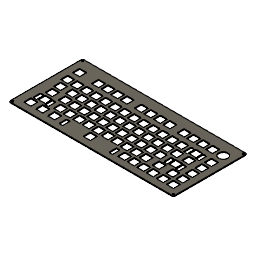
_Top_Mech_Case.fb088db0-0566-425f-93ac-fc1d6e48a953 (Autodesk Fusion 360 design; units mm, degrees)
part number: 2026-01-11-19-49-38-762
Autodesk Fusion 360 part; units mm, degrees
(part 1 of 3)
sketch "plate-2026-01-07T20_54_01.375Z" plane through (0, 0, 0) normal (0, 0, 1) x (1, 0, 0)
  line L0 (-11.2624, -135.013) -> (318.4436, -135.013)
  line L1 (318.4436, -135.013) -> (318.4436, 12.475)
  line L2 (318.4436, 12.475) -> (-11.2624, 12.475)
  line L3 (-11.2624, 12.475) -> (-11.2624, -135.013)
  line L4 (3.025, -7.287) -> (16.025, -7.287)
  line L5 (3.025, -21.287) -> (16.025, -21.287)
  line L6 (2.525, -7.787) -> (2.525, -20.787)
  line L7 (16.525, -7.787) -> (16.525, -20.787)
  arc A0 (3.025, -7.287) -> (2.525, -7.787) centre (3.025, -7.787) ccw
  arc A1 (16.525, -7.787) -> (16.025, -7.287) centre (16.025, -7.787) ccw
  arc A2 (2.525, -20.787) -> (3.025, -21.287) centre (3.025, -20.787) ccw
  arc A3 (16.025, -21.287) -> (16.525, -20.787) centre (16.025, -20.787) ccw
  line L8 (41.125, -7.287) -> (54.125, -7.287)
  line L9 (41.125, -21.287) -> (54.125, -21.287)
  line L10 (40.625, -7.787) -> (40.625, -20.787)
  line L11 (54.625, -7.787) -> (54.625, -20.787)
  arc A4 (41.125, -7.287) -> (40.625, -7.787) centre (41.125, -7.787) ccw
  arc A5 (54.625, -7.787) -> (54.125, -7.287) centre (54.125, -7.787) ccw
  arc A6 (40.625, -20.787) -> (41.125, -21.287) centre (41.125, -20.787) ccw
  arc A7 (54.125, -21.287) -> (54.625, -20.787) centre (54.125, -20.787) ccw
  line L12 (60.175, -7.287) -> (73.175, -7.287)
  line L13 (60.175, -21.287) -> (73.175, -21.287)
  line L14 (59.675, -7.787) -> (59.675, -20.787)
  line L15 (73.675, -7.787) -> (73.675, -20.787)
  arc A8 (60.175, -7.287) -> (59.675, -7.787) centre (60.175, -7.787) ccw
  arc A9 (73.675, -7.787) -> (73.175, -7.287) centre (73.175, -7.787) ccw
  arc A10 (59.675, -20.787) -> (60.175, -21.287) centre (60.175, -20.787) ccw
  arc A11 (73.175, -21.287) -> (73.675, -20.787) centre (73.175, -20.787) ccw
  line L16 (79.225, -7.287) -> (92.225, -7.287)
  line L17 (79.225, -21.287) -> (92.225, -21.287)
  line L18 (78.725, -7.787) -> (78.725, -20.787)
  line L19 (92.725, -7.787) -> (92.725, -20.787)
  arc A12 (79.225, -7.287) -> (78.725, -7.787) centre (79.225, -7.787) ccw
  arc A13 (92.725, -7.787) -> (92.225, -7.287) centre (92.225, -7.787) ccw
  arc A14 (78.725, -20.787) -> (79.225, -21.287) centre (79.225, -20.787) ccw
  arc A15 (92.225, -21.287) -> (92.725, -20.787) centre (92.225, -20.787) ccw
  line L20 (98.275, -7.287) -> (111.275, -7.287)
  line L21 (98.275, -21.287) -> (111.275, -21.287)
  line L22 (97.775, -7.787) -> (97.775, -20.787)
  line L23 (111.775, -7.787) -> (111.775, -20.787)
  arc A16 (98.275, -7.287) -> (97.775, -7.787) centre (98.275, -7.787) ccw
  arc A17 (111.775, -7.787) -> (111.275, -7.287) centre (111.275, -7.787) ccw
  arc A18 (97.775, -20.787) -> (98.275, -21.287) centre (98.275, -20.787) ccw
  arc A19 (111.275, -21.287) -> (111.775, -20.787) centre (111.275, -20.787) ccw
  line L24 (126.8501, -7.287) -> (139.8501, -7.287)
  line L25 (126.8501, -21.287) -> (139.8501, -21.287)
  line L26 (126.3501, -7.787) -> (126.3501, -20.787)
  line L27 (140.3501, -7.787) -> (140.3501, -20.787)
  arc A20 (126.8501, -7.287) -> (126.3501, -7.787) centre (126.8501, -7.787) ccw
  arc A21 (140.3501, -7.787) -> (139.8501, -7.287) centre (139.8501, -7.787) ccw
  arc A22 (126.3501, -20.787) -> (126.8501, -21.287) centre (126.8501, -20.787) ccw
  arc A23 (139.8501, -21.287) -> (140.3501, -20.787) centre (139.8501, -20.787) ccw
  line L28 (145.9001, -7.287) -> (158.9001, -7.287)
  line L29 (145.9001, -21.287) -> (158.9001, -21.287)
  line L30 (145.4001, -7.787) -> (145.4001, -20.787)
  line L31 (159.4001, -7.787) -> (159.4001, -20.787)
  arc A24 (145.9001, -7.287) -> (145.4001, -7.787) centre (145.9001, -7.787) ccw
  arc A25 (159.4001, -7.787) -> (158.9001, -7.287) centre (158.9001, -7.787) ccw
  arc A26 (145.4001, -20.787) -> (145.9001, -21.287) centre (145.9001, -20.787) ccw
  arc A27 (158.9001, -21.287) -> (159.4001, -20.787) centre (158.9001, -20.787) ccw
  line L32 (164.9501, -7.287) -> (177.9501, -7.287)
  line L33 (164.9501, -21.287) -> (177.9501, -21.287)
  line L34 (164.4501, -7.787) -> (164.4501, -20.787)
  line L35 (178.4501, -7.787) -> (178.4501, -20.787)
  arc A28 (164.9501, -7.287) -> (164.4501, -7.787) centre (164.9501, -7.787) ccw
  arc A29 (178.4501, -7.787) -> (177.9501, -7.287) centre (177.9501, -7.787) ccw
  arc A30 (164.4501, -20.787) -> (164.9501, -21.287) centre (164.9501, -20.787) ccw
  arc A31 (177.9501, -21.287) -> (178.4501, -20.787) centre (177.9501, -20.787) ccw
  line L36 (184.0001, -7.287) -> (197.0001, -7.287)
  line L37 (184.0001, -21.287) -> (197.0001, -21.287)
  line L38 (183.5001, -7.787) -> (183.5001, -20.787)
  line L39 (197.5001, -7.787) -> (197.5001, -20.787)
  arc A32 (184.0001, -7.287) -> (183.5001, -7.787) centre (184.0001, -7.787) ccw
  arc A33 (197.5001, -7.787) -> (197.0001, -7.287) centre (197.0001, -7.787) ccw
  arc A34 (183.5001, -20.787) -> (184.0001, -21.287) centre (184.0001, -20.787) ccw
  arc A35 (197.0001, -21.287) -> (197.5001, -20.787) centre (197.0001, -20.787) ccw
  line L40 (212.5752, -7.287) -> (225.5752, -7.287)
  line L41 (212.5752, -21.287) -> (225.5752, -21.287)
  line L42 (212.0752, -7.787) -> (212.0752, -20.787)
  line L43 (226.0752, -7.787) -> (226.0752, -20.787)
  arc A36 (212.5752, -7.287) -> (212.0752, -7.787) centre (212.5752, -7.787) ccw
  arc A37 (226.0752, -7.787) -> (225.5752, -7.287) centre (225.5752, -7.787) ccw
  arc A38 (212.0752, -20.787) -> (212.5752, -21.287) centre (212.5752, -20.787) ccw
  arc A39 (225.5752, -21.287) -> (226.0752, -20.787) centre (225.5752, -20.787) ccw
  line L44 (231.6252, -7.287) -> (244.6252, -7.287)
  line L45 (231.6253, -21.287) -> (244.6252, -21.287)
  line L46 (231.1252, -7.787) -> (231.1252, -20.787)
  line L47 (245.1252, -7.787) -> (245.1252, -20.787)
  arc A40 (231.6252, -7.287) -> (231.1252, -7.787) centre (231.6252, -7.787) ccw
  arc A41 (245.1252, -7.787) -> (244.6252, -7.287) centre (244.6252, -7.787) ccw
  arc A42 (231.1252, -20.787) -> (231.6253, -21.287) centre (231.6253, -20.787) ccw
  arc A43 (244.6252, -21.287) -> (245.1252, -20.787) centre (244.6252, -20.787) ccw
  line L48 (250.6752, -7.287) -> (263.6752, -7.287)
  line L49 (250.6753, -21.287) -> (263.6752, -21.287)
  line L50 (250.1752, -7.787) -> (250.1753, -20.787)
  line L51 (264.1753, -7.787) -> (264.1753, -20.787)
  arc A44 (250.6752, -7.287) -> (250.1752, -7.787) centre (250.6752, -7.787) ccw
  arc A45 (264.1753, -7.787) -> (263.6752, -7.287) centre (263.6752, -7.787) ccw
  arc A46 (250.1753, -20.787) -> (250.6753, -21.287) centre (250.6753, -20.787) ccw
  arc A47 (263.6752, -21.287) -> (264.1753, -20.787) centre (263.6752, -20.787) ccw
  line L52 (269.7253, -7.287) -> (282.7252, -7.287)
  line L53 (269.7253, -21.287) -> (282.7252, -21.287)
  line L54 (269.2252, -7.787) -> (269.2253, -20.787)
  line L55 (283.2253, -7.787) -> (283.2253, -20.787)
  arc A48 (269.7253, -7.287) -> (269.2252, -7.787) centre (269.7253, -7.787) ccw
  arc A49 (283.2253, -7.787) -> (282.7252, -7.287) centre (282.7252, -7.787) ccw
  arc A50 (269.2253, -20.787) -> (269.7253, -21.287) centre (269.7253, -20.787) ccw
  arc A51 (282.7252, -21.287) -> (283.2253, -20.787) centre (282.7252, -20.787) ccw
  line L56 (3.025, -31.1) -> (16.025, -31.1)
  line L57 (3.025, -45.1) -> (16.025, -45.1)
  line L58 (2.525, -31.6) -> (2.525, -44.6)
  line L59 (16.525, -31.6) -> (16.525, -44.6)
  arc A52 (3.025, -31.1) -> (2.525, -31.6) centre (3.025, -31.6) ccw
  arc A53 (16.525, -31.6) -> (16.025, -31.1) centre (16.025, -31.6) ccw
  arc A54 (2.525, -44.6) -> (3.025, -45.1) centre (3.025, -44.6) ccw
  arc A55 (16.025, -45.1) -> (16.525, -44.6) centre (16.025, -44.6) ccw
  line L60 (22.075, -31.1) -> (35.075, -31.1)
  line L61 (22.075, -45.1) -> (35.075, -45.1)
  line L62 (21.575, -31.6) -> (21.575, -44.6)
  line L63 (35.575, -31.6) -> (35.575, -44.6)
  arc A56 (22.075, -31.1) -> (21.575, -31.6) centre (22.075, -31.6) ccw
  arc A57 (35.575, -31.6) -> (35.075, -31.1) centre (35.075, -31.6) ccw
  arc A58 (21.575, -44.6) -> (22.075, -45.1) centre (22.075, -44.6) ccw
  arc A59 (35.075, -45.1) -> (35.575, -44.6) centre (35.075, -44.6) ccw
  line L64 (41.125, -31.1) -> (54.125, -31.1)
  line L65 (41.125, -45.1) -> (54.125, -45.1)
  line L66 (40.625, -31.6) -> (40.625, -44.6)
  line L67 (54.625, -31.6) -> (54.625, -44.6)
  arc A60 (41.125, -31.1) -> (40.625, -31.6) centre (41.125, -31.6) ccw
  arc A61 (54.625, -31.6) -> (54.125, -31.1) centre (54.125, -31.6) ccw
  arc A62 (40.625, -44.6) -> (41.125, -45.1) centre (41.125, -44.6) ccw
  arc A63 (54.125, -45.1) -> (54.625, -44.6) centre (54.125, -44.6) ccw
  line L68 (60.175, -31.1) -> (73.175, -31.1)
  line L69 (60.175, -45.1) -> (73.175, -45.1)
  line L70 (59.675, -31.6) -> (59.675, -44.6)
  line L71 (73.675, -31.6) -> (73.675, -44.6)
  arc A64 (60.175, -31.1) -> (59.675, -31.6) centre (60.175, -31.6) ccw
  arc A65 (73.675, -31.6) -> (73.175, -31.1) centre (73.175, -31.6) ccw
  arc A66 (59.675, -44.6) -> (60.175, -45.1) centre (60.175, -44.6) ccw
  arc A67 (73.175, -45.1) -> (73.675, -44.6) centre (73.175, -44.6) ccw
  line L72 (79.225, -31.1) -> (92.225, -31.1)
  line L73 (79.225, -45.1) -> (92.225, -45.1)
  line L74 (78.725, -31.6) -> (78.725, -44.6)
  line L75 (92.725, -31.6) -> (92.725, -44.6)
  arc A68 (79.225, -31.1) -> (78.725, -31.6) centre (79.225, -31.6) ccw
  arc A69 (92.725, -31.6) -> (92.225, -31.1) centre (92.225, -31.6) ccw
  arc A70 (78.725, -44.6) -> (79.225, -45.1) centre (79.225, -44.6) ccw
  arc A71 (92.225, -45.1) -> (92.725, -44.6) centre (92.225, -44.6) ccw
  line L76 (98.275, -31.1) -> (111.275, -31.1)
  line L77 (98.275, -45.1) -> (111.275, -45.1)
  line L78 (97.775, -31.6) -> (97.775, -44.6)
  line L79 (111.775, -31.6) -> (111.775, -44.6)
  arc A72 (98.275, -31.1) -> (97.775, -31.6) centre (98.275, -31.6) ccw
  arc A73 (111.775, -31.6) -> (111.275, -31.1) centre (111.275, -31.6) ccw
  arc A74 (97.775, -44.6) -> (98.275, -45.1) centre (98.275, -44.6) ccw
  arc A75 (111.275, -45.1) -> (111.775, -44.6) centre (111.275, -44.6) ccw
  line L80 (117.325, -31.1) -> (130.325, -31.1)
  line L81 (117.325, -45.1) -> (130.325, -45.1)
  line L82 (116.825, -31.6) -> (116.825, -44.6)
  line L83 (130.825, -31.6) -> (130.825, -44.6)
  arc A76 (117.325, -31.1) -> (116.825, -31.6) centre (117.325, -31.6) ccw
  arc A77 (130.825, -31.6) -> (130.325, -31.1) centre (130.325, -31.6) ccw
  arc A78 (116.825, -44.6) -> (117.325, -45.1) centre (117.325, -44.6) ccw
  arc A79 (130.325, -45.1) -> (130.825, -44.6) centre (130.325, -44.6) ccw
  line L84 (136.375, -31.1) -> (149.375, -31.1)
  line L85 (136.375, -45.1) -> (149.375, -45.1)
  line L86 (135.875, -31.6) -> (135.875, -44.6)
  line L87 (149.875, -31.6) -> (149.875, -44.6)
  arc A80 (136.375, -31.1) -> (135.875, -31.6) centre (136.375, -31.6) ccw
  arc A81 (149.875, -31.6) -> (149.375, -31.1) centre (149.375, -31.6) ccw
  arc A82 (135.875, -44.6) -> (136.375, -45.1) centre (136.375, -44.6) ccw
  arc A83 (149.375, -45.1) -> (149.875, -44.6) centre (149.375, -44.6) ccw
  line L88 (155.425, -31.1) -> (168.425, -31.1)
  line L89 (155.425, -45.1) -> (168.425, -45.1)
  line L90 (154.925, -31.6) -> (154.925, -44.6)
  line L91 (168.925, -31.6) -> (168.925, -44.6)
  arc A84 (155.425, -31.1) -> (154.925, -31.6) centre (155.425, -31.6) ccw
  arc A85 (168.925, -31.6) -> (168.425, -31.1) centre (168.425, -31.6) ccw
  arc A86 (154.925, -44.6) -> (155.425, -45.1) centre (155.425, -44.6) ccw
  arc A87 (168.425, -45.1) -> (168.925, -44.6) centre (168.425, -44.6) ccw
  line L92 (174.475, -31.1) -> (187.475, -31.1)
  line L93 (174.475, -45.1) -> (187.475, -45.1)
  line L94 (173.975, -31.6) -> (173.975, -44.6)
  line L95 (187.975, -31.6) -> (187.975, -44.6)
  arc A88 (174.475, -31.1) -> (173.975, -31.6) centre (174.475, -31.6) ccw
  arc A89 (187.975, -31.6) -> (187.475, -31.1) centre (187.475, -31.6) ccw
  arc A90 (173.975, -44.6) -> (174.475, -45.1) centre (174.475, -44.6) ccw
  arc A91 (187.475, -45.1) -> (187.975, -44.6) centre (187.475, -44.6) ccw
  line L96 (193.525, -31.1) -> (206.525, -31.1)
  line L97 (193.525, -45.1) -> (206.525, -45.1)
  line L98 (193.025, -31.6) -> (193.025, -44.6)
  line L99 (207.025, -31.6) -> (207.025, -44.6)
  arc A92 (193.525, -31.1) -> (193.025, -31.6) centre (193.525, -31.6) ccw
  arc A93 (207.025, -31.6) -> (206.525, -31.1) centre (206.525, -31.6) ccw
  arc A94 (193.025, -44.6) -> (193.525, -45.1) centre (193.525, -44.6) ccw
  arc A95 (206.525, -45.1) -> (207.025, -44.6) centre (206.525, -44.6) ccw
  line L100 (212.575, -31.1) -> (225.575, -31.1)
  line L101 (212.575, -45.1) -> (225.575, -45.1)
  line L102 (212.075, -31.6) -> (212.075, -44.6)
  line L103 (226.075, -31.6) -> (226.075, -44.6)
  arc A96 (212.575, -31.1) -> (212.075, -31.6) centre (212.575, -31.6) ccw
  arc A97 (226.075, -31.6) -> (225.575, -31.1) centre (225.575, -31.6) ccw
  arc A98 (212.075, -44.6) -> (212.575, -45.1) centre (212.575, -44.6) ccw
  arc A99 (225.575, -45.1) -> (226.075, -44.6) centre (225.575, -44.6) ccw
  line L104 (231.625, -31.1) -> (244.625, -31.1)
  line L105 (231.625, -45.1) -> (244.625, -45.1)
  line L106 (231.125, -31.6) -> (231.125, -44.6)
  line L107 (245.125, -31.6) -> (245.125, -44.6)
  arc A100 (231.625, -31.1) -> (231.125, -31.6) centre (231.625, -31.6) ccw
  arc A101 (245.125, -31.6) -> (244.625, -31.1) centre (244.625, -31.6) ccw
  arc A102 (231.125, -44.6) -> (231.625, -45.1) centre (231.625, -44.6) ccw
  arc A103 (244.625, -45.1) -> (245.125, -44.6) centre (244.625, -44.6) ccw
  line L108 (260.2, -31.1) -> (273.2, -31.1)
  line L109 (260.2, -45.1) -> (273.2, -45.1)
  line L110 (259.7, -31.6) -> (259.7, -44.6)
  line L111 (273.7, -31.6) -> (273.7, -44.6)
  arc A104 (260.2, -31.1) -> (259.7, -31.6) centre (260.2, -31.6) ccw
  arc A105 (273.7, -31.6) -> (273.2, -31.1) centre (273.2, -31.6) ccw
  arc A106 (259.7, -44.6) -> (260.2, -45.1) centre (260.2, -44.6) ccw
  arc A107 (273.2, -45.1) -> (273.7, -44.6) centre (273.2, -44.6) ccw
  line L112 (251.762, -32.1) -> (257.762, -32.1)
  line L113 (251.762, -47.1) -> (257.762, -47.1)
  line L114 (251.262, -32.6) -> (251.262, -46.6)
  line L115 (258.262, -32.6) -> (258.262, -46.6)
  arc A108 (251.762, -32.1) -> (251.262, -32.6) centre (251.762, -32.6) ccw
  arc A109 (258.262, -32.6) -> (257.762, -32.1) centre (257.762, -32.6) ccw
  arc A110 (251.262, -46.6) -> (251.762, -47.1) centre (251.762, -46.6) ccw
  arc A111 (257.762, -47.1) -> (258.262, -46.6) centre (257.762, -46.6) ccw
  line L116 (275.638, -32.1) -> (281.638, -32.1)
  line L117 (275.638, -47.1) -> (281.638, -47.1)
  line L118 (275.138, -32.6) -> (275.138, -46.6)
  line L119 (282.138, -32.6) -> (282.138, -46.6)
  arc A112 (275.638, -32.1) -> (275.138, -32.6) centre (275.638, -32.6) ccw
  arc A113 (282.138, -32.6) -> (281.638, -32.1) centre (281.638, -32.6) ccw
  arc A114 (275.138, -46.6) -> (275.638, -47.1) centre (275.638, -46.6) ccw
  arc A115 (281.638, -47.1) -> (282.138, -46.6) centre (281.638, -46.6) ccw
  line L120 (291.1562, -31.1) -> (304.1562, -31.1)
  line L121 (291.1562, -45.1) -> (304.1562, -45.1)
  line L122 (290.6562, -31.6) -> (290.6562, -44.6)
  line L123 (304.6562, -31.6) -> (304.6562, -44.6)
  arc A116 (291.1562, -31.1) -> (290.6562, -31.6) centre (291.1562, -31.6) ccw
  arc A117 (304.6562, -31.6) -> (304.1562, -31.1) centre (304.1562, -31.6) ccw
  arc A118 (290.6562, -44.6) -> (291.1562, -45.1) centre (291.1562, -44.6) ccw
  arc A119 (304.1562, -45.1) -> (304.6562, -44.6) centre (304.1562, -44.6) ccw
  line L124 (7.7875, -50.15) -> (20.7875, -50.15)
  line L125 (7.7875, -64.15) -> (20.7875, -64.15)
  line L126 (7.2875, -50.65) -> (7.2875, -63.65)
  line L127 (21.2875, -50.65) -> (21.2875, -63.65)
  arc A120 (7.7875, -50.15) -> (7.2875, -50.65) centre (7.7875, -50.65) ccw
  arc A121 (21.2875, -50.65) -> (20.7875, -50.15) centre (20.7875, -50.65) ccw
  arc A122 (7.2875, -63.65) -> (7.7875, -64.15) centre (7.7875, -63.65) ccw
  arc A123 (20.7875, -64.15) -> (21.2875, -63.65) centre (20.7875, -63.65) ccw
  line L128 (31.6, -50.15) -> (44.6, -50.15)
  line L129 (31.6, -64.15) -> (44.6, -64.15)
  line L130 (31.1, -50.65) -> (31.1, -63.65)
  line L131 (45.1, -50.65) -> (45.1, -63.65)
  arc A124 (31.6, -50.15) -> (31.1, -50.65) centre (31.6, -50.65) ccw
  arc A125 (45.1, -50.65) -> (44.6, -50.15) centre (44.6, -50.65) ccw
  arc A126 (31.1, -63.65) -> (31.6, -64.15) centre (31.6, -63.65) ccw
  arc A127 (44.6, -64.15) -> (45.1, -63.65) centre (44.6, -63.65) ccw
  line L132 (50.65, -50.15) -> (63.65, -50.15)
  line L133 (50.65, -64.15) -> (63.65, -64.15)
  line L134 (50.15, -50.65) -> (50.15, -63.65)
  line L135 (64.15, -50.65) -> (64.15, -63.65)
  arc A128 (50.65, -50.15) -> (50.15, -50.65) centre (50.65, -50.65) ccw
  arc A129 (64.15, -50.65) -> (63.65, -50.15) centre (63.65, -50.65) ccw
  arc A130 (50.15, -63.65) -> (50.65, -64.15) centre (50.65, -63.65) ccw
  arc A131 (63.65, -64.15) -> (64.15, -63.65) centre (63.65, -63.65) ccw
  line L136 (69.7, -50.15) -> (82.7, -50.15)
  line L137 (69.7, -64.15) -> (82.7, -64.15)
  line L138 (69.2, -50.65) -> (69.2, -63.65)
  line L139 (83.2, -50.65) -> (83.2, -63.65)
  arc A132 (69.7, -50.15) -> (69.2, -50.65) centre (69.7, -50.65) ccw
  arc A133 (83.2, -50.65) -> (82.7, -50.15) centre (82.7, -50.65) ccw
  arc A134 (69.2, -63.65) -> (69.7, -64.15) centre (69.7, -63.65) ccw
  arc A135 (82.7, -64.15) -> (83.2, -63.65) centre (82.7, -63.65) ccw
  line L140 (88.75, -50.15) -> (101.75, -50.15)
  line L141 (88.75, -64.15) -> (101.75, -64.15)
  line L142 (88.25, -50.65) -> (88.25, -63.65)
  line L143 (102.25, -50.65) -> (102.25, -63.65)
  arc A136 (88.75, -50.15) -> (88.25, -50.65) centre (88.75, -50.65) ccw
  arc A137 (102.25, -50.65) -> (101.75, -50.15) centre (101.75, -50.65) ccw
  arc A138 (88.25, -63.65) -> (88.75, -64.15) centre (88.75, -63.65) ccw
  arc A139 (101.75, -64.15) -> (102.25, -63.65) centre (101.75, -63.65) ccw
  line L144 (107.8, -50.15) -> (120.8, -50.15)
  line L145 (107.8, -64.15) -> (120.8, -64.15)
  line L146 (107.3, -50.65) -> (107.3, -63.65)
  line L147 (121.3, -50.65) -> (121.3, -63.65)
  arc A140 (107.8, -50.15) -> (107.3, -50.65) centre (107.8, -50.65) ccw
  arc A141 (121.3, -50.65) -> (120.8, -50.15) centre (120.8, -50.65) ccw
  arc A142 (107.3, -63.65) -> (107.8, -64.15) centre (107.8, -63.65) ccw
  arc A143 (120.8, -64.15) -> (121.3, -63.65) centre (120.8, -63.65) ccw
  line L148 (126.85, -50.15) -> (139.85, -50.15)
  line L149 (126.85, -64.15) -> (139.85, -64.15)
  line L150 (126.35, -50.65) -> (126.35, -63.65)
  line L151 (140.35, -50.65) -> (140.35, -63.65)
  arc A144 (126.85, -50.15) -> (126.35, -50.65) centre (126.85, -50.65) ccw
  arc A145 (140.35, -50.65) -> (139.85, -50.15) centre (139.85, -50.65) ccw
  arc A146 (126.35, -63.65) -> (126.85, -64.15) centre (126.85, -63.65) ccw
  arc A147 (139.85, -64.15) -> (140.35, -63.65) centre (139.85, -63.65) ccw
  line L152 (145.9, -50.15) -> (158.9, -50.15)
  line L153 (145.9, -64.15) -> (158.9, -64.15)
  line L154 (145.4, -50.65) -> (145.4, -63.65)
  line L155 (159.4, -50.65) -> (159.4, -63.65)
  arc A148 (145.9, -50.15) -> (145.4, -50.65) centre (145.9, -50.65) ccw
  arc A149 (159.4, -50.65) -> (158.9, -50.15) centre (158.9, -50.65) ccw
  arc A150 (145.4, -63.65) -> (145.9, -64.15) centre (145.9, -63.65) ccw
  arc A151 (158.9, -64.15) -> (159.4, -63.65) centre (158.9, -63.65) ccw
  line L156 (164.95, -50.15) -> (177.95, -50.15)
  line L157 (164.95, -64.15) -> (177.95, -64.15)
  line L158 (164.45, -50.65) -> (164.45, -63.65)
  line L159 (178.45, -50.65) -> (178.45, -63.65)
  arc A152 (164.95, -50.15) -> (164.45, -50.65) centre (164.95, -50.65) ccw
  arc A153 (178.45, -50.65) -> (177.95, -50.15) centre (177.95, -50.65) ccw
  arc A154 (164.45, -63.65) -> (164.95, -64.15) centre (164.95, -63.65) ccw
  arc A155 (177.95, -64.15) -> (178.45, -63.65) centre (177.95, -63.65) ccw
  line L160 (184, -50.15) -> (197, -50.15)
  line L161 (184, -64.15) -> (197, -64.15)
  line L162 (183.5, -50.65) -> (183.5, -63.65)
  line L163 (197.5, -50.65) -> (197.5, -63.65)
  arc A156 (184, -50.15) -> (183.5, -50.65) centre (184, -50.65) ccw
  arc A157 (197.5, -50.65) -> (197, -50.15) centre (197, -50.65) ccw
  arc A158 (183.5, -63.65) -> (184, -64.15) centre (184, -63.65) ccw
  arc A159 (197, -64.15) -> (197.5, -63.65) centre (197, -63.65) ccw
  line L164 (203.05, -50.15) -> (216.05, -50.15)
  line L165 (203.05, -64.15) -> (216.05, -64.15)
  line L166 (202.55, -50.65) -> (202.55, -63.65)
  line L167 (216.55, -50.65) -> (216.55, -63.65)
  arc A160 (203.05, -50.15) -> (202.55, -50.65) centre (203.05, -50.65) ccw
  arc A161 (216.55, -50.65) -> (216.05, -50.15) centre (216.05, -50.65) ccw
  arc A162 (202.55, -63.65) -> (203.05, -64.15) centre (203.05, -63.65) ccw
  arc A163 (216.05, -64.15) -> (216.55, -63.65) centre (216.05, -63.65) ccw
  line L168 (222.1, -50.15) -> (235.1, -50.15)
  line L169 (222.1, -64.15) -> (235.1, -64.15)
  line L170 (221.6, -50.65) -> (221.6, -63.65)
  line L171 (235.6, -50.65) -> (235.6, -63.65)
  arc A164 (222.1, -50.15) -> (221.6, -50.65) centre (222.1, -50.65) ccw
  arc A165 (235.6, -50.65) -> (235.1, -50.15) centre (235.1, -50.65) ccw
  arc A166 (221.6, -63.65) -> (222.1, -64.15) centre (222.1, -63.65) ccw
  arc A167 (235.1, -64.15) -> (235.6, -63.65) centre (235.1, -63.65) ccw
  line L172 (241.15, -50.15) -> (254.15, -50.15)
  line L173 (241.15, -64.15) -> (254.15, -64.15)
  line L174 (240.65, -50.65) -> (240.65, -63.65)
  line L175 (254.65, -50.65) -> (254.65, -63.65)
  arc A168 (241.15, -50.15) -> (240.65, -50.65) centre (241.15, -50.65) ccw
  arc A169 (254.65, -50.65) -> (254.15, -50.15) centre (254.15, -50.65) ccw
  arc A170 (240.65, -63.65) -> (241.15, -64.15) centre (241.15, -63.65) ccw
  arc A171 (254.15, -64.15) -> (254.65, -63.65) centre (254.15, -63.65) ccw
  line L176 (264.9625, -50.15) -> (277.9625, -50.15)
  line L177 (264.9625, -64.15) -> (277.9625, -64.15)
  line L178 (264.4625, -50.65) -> (264.4625, -63.65)
  line L179 (278.4625, -50.65) -> (278.4625, -63.65)
  arc A172 (264.9625, -50.15) -> (264.4625, -50.65) centre (264.9625, -50.65) ccw
  arc A173 (278.4625, -50.65) -> (277.9625, -50.15) centre (277.9625, -50.65) ccw
  arc A174 (264.4625, -63.65) -> (264.9625, -64.15) centre (264.9625, -63.65) ccw
  arc A175 (277.9625, -64.15) -> (278.4625, -63.65) centre (277.9625, -63.65) ccw
  line L180 (291.1562, -50.15) -> (304.1562, -50.15)
  line L181 (291.1562, -64.15) -> (304.1562, -64.15)
  line L182 (290.6562, -50.65) -> (290.6562, -63.65)
  line L183 (304.6562, -50.65) -> (304.6562, -63.65)
  arc A176 (291.1562, -50.15) -> (290.6562, -50.65) centre (291.1562, -50.65) ccw
  arc A177 (304.6562, -50.65) -> (304.1562, -50.15) centre (304.1562, -50.65) ccw
  arc A178 (290.6562, -63.65) -> (291.1562, -64.15) centre (291.1562, -63.65) ccw
  arc A179 (304.1562, -64.15) -> (304.6562, -63.65) centre (304.1562, -63.65) ccw
  line L184 (10.1687, -69.2) -> (23.1687, -69.2)
  line L185 (10.1687, -83.2) -> (23.1687, -83.2)
  line L186 (9.6687, -69.7) -> (9.6687, -82.7)
  line L187 (23.6687, -69.7) -> (23.6687, -82.7)
  arc A180 (10.1687, -69.2) -> (9.6688, -69.7) centre (10.1687, -69.7) ccw
  arc A181 (23.6687, -69.7) -> (23.1687, -69.2) centre (23.1687, -69.7) ccw
  arc A182 (9.6687, -82.7) -> (10.1687, -83.2) centre (10.1687, -82.7) ccw
  arc A183 (23.1687, -83.2) -> (23.6687, -82.7) centre (23.1687, -82.7) ccw
  line L188 (36.3625, -69.2) -> (49.3625, -69.2)
  line L189 (36.3625, -83.2) -> (49.3625, -83.2)
  line L190 (35.8625, -69.7) -> (35.8625, -82.7)
  line L191 (49.8625, -69.7) -> (49.8625, -82.7)
  arc A184 (36.3625, -69.2) -> (35.8625, -69.7) centre (36.3625, -69.7) ccw
  arc A185 (49.8625, -69.7) -> (49.3625, -69.2) centre (49.3625, -69.7) ccw
  arc A186 (35.8625, -82.7) -> (36.3625, -83.2) centre (36.3625, -82.7) ccw
  arc A187 (49.3625, -83.2) -> (49.8625, -82.7) centre (49.3625, -82.7) ccw
  line L192 (55.4125, -69.2) -> (68.4125, -69.2)
  line L193 (55.4125, -83.2) -> (68.4125, -83.2)
  line L194 (54.9125, -69.7) -> (54.9125, -82.7)
  line L195 (68.9125, -69.7) -> (68.9125, -82.7)
  arc A188 (55.4125, -69.2) -> (54.9125, -69.7) centre (55.4125, -69.7) ccw
  arc A189 (68.9125, -69.7) -> (68.4125, -69.2) centre (68.4125, -69.7) ccw
  arc A190 (54.9125, -82.7) -> (55.4125, -83.2) centre (55.4125, -82.7) ccw
  arc A191 (68.4125, -83.2) -> (68.9125, -82.7) centre (68.4125, -82.7) ccw
  line L196 (74.4625, -69.2) -> (87.4625, -69.2)
  line L197 (74.4625, -83.2) -> (87.4625, -83.2)
  line L198 (73.9625, -69.7) -> (73.9625, -82.7)
  line L199 (87.9625, -69.7) -> (87.9625, -82.7)
  arc A192 (74.4625, -69.2) -> (73.9625, -69.7) centre (74.4625, -69.7) ccw
  arc A193 (87.9625, -69.7) -> (87.4625, -69.2) centre (87.4625, -69.7) ccw
  arc A194 (73.9625, -82.7) -> (74.4625, -83.2) centre (74.4625, -82.7) ccw
  arc A195 (87.4625, -83.2) -> (87.9625, -82.7) centre (87.4625, -82.7) ccw
  line L200 (93.5125, -69.2) -> (106.5125, -69.2)
  line L201 (93.5125, -83.2) -> (106.5125, -83.2)
  line L202 (93.0125, -69.7) -> (93.0125, -82.7)
  line L203 (107.0125, -69.7) -> (107.0125, -82.7)
  arc A196 (93.5125, -69.2) -> (93.0125, -69.7) centre (93.5125, -69.7) ccw
  arc A197 (107.0125, -69.7) -> (106.5125, -69.2) centre (106.5125, -69.7) ccw
  arc A198 (93.0125, -82.7) -> (93.5125, -83.2) centre (93.5125, -82.7) ccw
  arc A199 (106.5125, -83.2) -> (107.0125, -82.7) centre (106.5125, -82.7) ccw
  line L204 (112.5625, -69.2) -> (125.5625, -69.2)
  line L205 (112.5625, -83.2) -> (125.5625, -83.2)
  line L206 (112.0625, -69.7) -> (112.0625, -82.7)
  line L207 (126.0625, -69.7) -> (126.0625, -82.7)
  arc A200 (112.5625, -69.2) -> (112.0625, -69.7) centre (112.5625, -69.7) ccw
  arc A201 (126.0625, -69.7) -> (125.5625, -69.2) centre (125.5625, -69.7) ccw
  arc A202 (112.0625, -82.7) -> (112.5625, -83.2) centre (112.5625, -82.7) ccw
  arc A203 (125.5625, -83.2) -> (126.0625, -82.7) centre (125.5625, -82.7) ccw
  line L208 (131.6125, -69.2) -> (144.6125, -69.2)
  line L209 (131.6125, -83.2) -> (144.6125, -83.2)
  line L210 (131.1125, -69.7) -> (131.1125, -82.7)
  line L211 (145.1125, -69.7) -> (145.1125, -82.7)
  arc A204 (131.6125, -69.2) -> (131.1125, -69.7) centre (131.6125, -69.7) ccw
  arc A205 (145.1125, -69.7) -> (144.6125, -69.2) centre (144.6125, -69.7) ccw
  arc A206 (131.1125, -82.7) -> (131.6125, -83.2) centre (131.6125, -82.7) ccw
  arc A207 (144.6125, -83.2) -> (145.1125, -82.7) centre (144.6125, -82.7) ccw
  line L212 (150.6625, -69.2) -> (163.6625, -69.2)
  line L213 (150.6625, -83.2) -> (163.6625, -83.2)
  line L214 (150.1625, -69.7) -> (150.1625, -82.7)
  line L215 (164.1625, -69.7) -> (164.1625, -82.7)
  arc A208 (150.6625, -69.2) -> (150.1625, -69.7) centre (150.6625, -69.7) ccw
  arc A209 (164.1625, -69.7) -> (163.6625, -69.2) centre (163.6625, -69.7) ccw
  arc A210 (150.1625, -82.7) -> (150.6625, -83.2) centre (150.6625, -82.7) ccw
  arc A211 (163.6625, -83.2) -> (164.1625, -82.7) centre (163.6625, -82.7) ccw
  line L216 (169.7125, -69.2) -> (182.7125, -69.2)
  line L217 (169.7125, -83.2) -> (182.7125, -83.2)
  line L218 (169.2125, -69.7) -> (169.2125, -82.7)
  line L219 (183.2125, -69.7) -> (183.2125, -82.7)
  arc A212 (169.7125, -69.2) -> (169.2125, -69.7) centre (169.7125, -69.7) ccw
  arc A213 (183.2125, -69.7) -> (182.7125, -69.2) centre (182.7125, -69.7) ccw
  arc A214 (169.2125, -82.7) -> (169.7125, -83.2) centre (169.7125, -82.7) ccw
  arc A215 (182.7125, -83.2) -> (183.2125, -82.7) centre (182.7125, -82.7) ccw
  line L220 (188.7625, -69.2) -> (201.7625, -69.2)
  line L221 (188.7625, -83.2) -> (201.7625, -83.2)
  line L222 (188.2625, -69.7) -> (188.2625, -82.7)
  line L223 (202.2625, -69.7) -> (202.2625, -82.7)
  arc A216 (188.7625, -69.2) -> (188.2625, -69.7) centre (188.7625, -69.7) ccw
  arc A217 (202.2625, -69.7) -> (201.7625, -69.2) centre (201.7625, -69.7) ccw
  arc A218 (188.2625, -82.7) -> (188.7625, -83.2) centre (188.7625, -82.7) ccw
  arc A219 (201.7625, -83.2) -> (202.2625, -82.7) centre (201.7625, -82.7) ccw
  line L224 (207.8125, -69.2) -> (220.8125, -69.2)
  line L225 (207.8125, -83.2) -> (220.8125, -83.2)
  line L226 (207.3125, -69.7) -> (207.3125, -82.7)
  line L227 (221.3125, -69.7) -> (221.3125, -82.7)
  arc A220 (207.8125, -69.2) -> (207.3125, -69.7) centre (207.8125, -69.7) ccw
  arc A221 (221.3125, -69.7) -> (220.8125, -69.2) centre (220.8125, -69.7) ccw
  arc A222 (207.3125, -82.7) -> (207.8125, -83.2) centre (207.8125, -82.7) ccw
  arc A223 (220.8125, -83.2) -> (221.3125, -82.7) centre (220.8125, -82.7) ccw
  line L228 (226.8625, -69.2) -> (239.8625, -69.2)
  line L229 (226.8625, -83.2) -> (239.8625, -83.2)
  line L230 (226.3625, -69.7) -> (226.3625, -82.7)
  line L231 (240.3625, -69.7) -> (240.3625, -82.7)
  arc A224 (226.8625, -69.2) -> (226.3625, -69.7) centre (226.8625, -69.7) ccw
  arc A225 (240.3625, -69.7) -> (239.8625, -69.2) centre (239.8625, -69.7) ccw
  arc A226 (226.3625, -82.7) -> (226.8625, -83.2) centre (226.8625, -82.7) ccw
  arc A227 (239.8625, -83.2) -> (240.3625, -82.7) centre (239.8625, -82.7) ccw
  line L232 (257.8188, -69.2) -> (270.8188, -69.2)
  line L233 (257.8188, -83.2) -> (270.8188, -83.2)
  line L234 (257.3188, -69.7) -> (257.3188, -82.7)
  line L235 (271.3188, -69.7) -> (271.3188, -82.7)
  arc A228 (257.8188, -69.2) -> (257.3188, -69.7) centre (257.8188, -69.7) ccw
  arc A229 (271.3188, -69.7) -> (270.8188, -69.2) centre (270.8188, -69.7) ccw
  arc A230 (257.3188, -82.7) -> (257.8188, -83.2) centre (257.8188, -82.7) ccw
  arc A231 (270.8188, -83.2) -> (271.3188, -82.7) centre (270.8188, -82.7) ccw
  line L236 (249.3808, -70.2) -> (255.3808, -70.2)
  line L237 (249.3808, -85.2) -> (255.3808, -85.2)
  line L238 (248.8808, -70.7) -> (248.8808, -84.7)
  line L239 (255.8808, -70.7) -> (255.8808, -84.7)
  arc A232 (249.3808, -70.2) -> (248.8808, -70.7) centre (249.3808, -70.7) ccw
  arc A233 (255.8808, -70.7) -> (255.3808, -70.2) centre (255.3808, -70.7) ccw
  arc A234 (248.8808, -84.7) -> (249.3808, -85.2) centre (249.3808, -84.7) ccw
  arc A235 (255.3808, -85.2) -> (255.8808, -84.7) centre (255.3808, -84.7) ccw
  line L240 (273.2568, -70.2) -> (279.2568, -70.2)
  line L241 (273.2568, -85.2) -> (279.2568, -85.2)
  line L242 (272.7568, -70.7) -> (272.7568, -84.7)
  line L243 (279.7568, -70.7) -> (279.7568, -84.7)
  arc A236 (273.2568, -70.2) -> (272.7568, -70.7) centre (273.2568, -70.7) ccw
  arc A237 (279.7568, -70.7) -> (279.2568, -70.2) centre (279.2568, -70.7) ccw
  arc A238 (272.7568, -84.7) -> (273.2568, -85.2) centre (273.2568, -84.7) ccw
  arc A239 (279.2568, -85.2) -> (279.7568, -84.7) centre (279.2568, -84.7) ccw
  line L244 (291.1562, -69.2) -> (304.1562, -69.2)
  line L245 (291.1562, -83.2) -> (304.1562, -83.2)
  line L246 (290.6562, -69.7) -> (290.6562, -82.7)
  line L247 (304.6562, -69.7) -> (304.6562, -82.7)
  arc A240 (291.1562, -69.2) -> (290.6562, -69.7) centre (291.1562, -69.7) ccw
  arc A241 (304.6562, -69.7) -> (304.1562, -69.2) centre (304.1562, -69.7) ccw
  arc A242 (290.6562, -82.7) -> (291.1562, -83.2) centre (291.1562, -82.7) ccw
  arc A243 (304.1562, -83.2) -> (304.6562, -82.7) centre (304.1562, -82.7) ccw
  line L248 (14.9313, -88.25) -> (27.9312, -88.25)
  line L249 (14.9313, -102.25) -> (27.9312, -102.25)
  line L250 (14.4313, -88.75) -> (14.4313, -101.75)
  line L251 (28.4313, -88.75) -> (28.4313, -101.75)
  arc A244 (14.9313, -88.25) -> (14.4313, -88.75) centre (14.9313, -88.75) ccw
  arc A245 (28.4313, -88.75) -> (27.9312, -88.25) centre (27.9312, -88.75) ccw
  arc A246 (14.4313, -101.75) -> (14.9313, -102.25) centre (14.9313, -101.75) ccw
  arc A247 (27.9312, -102.25) -> (28.4313, -101.75) centre (27.9312, -101.75) ccw
  line L252 (6.4933, -89.25) -> (12.4932, -89.25)
  line L253 (6.4933, -104.25) -> (12.4932, -104.25)
  line L254 (5.9932, -89.75) -> (5.9932, -103.75)
  line L255 (12.9932, -89.75) -> (12.9932, -103.75)
  arc A248 (6.4933, -89.25) -> (5.9933, -89.75) centre (6.4933, -89.75) ccw
  arc A249 (12.9932, -89.75) -> (12.4932, -89.25) centre (12.4932, -89.75) ccw
  arc A250 (5.9932, -103.75) -> (6.4933, -104.25) centre (6.4933, -103.75) ccw
  arc A251 (12.4932, -104.25) -> (12.9933, -103.75) centre (12.4932, -103.75) ccw
  line L256 (30.3693, -89.25) -> (36.3693, -89.25)
  line L257 (30.3693, -104.25) -> (36.3693, -104.25)
  line L258 (29.8693, -89.75) -> (29.8693, -103.75)
  line L259 (36.8693, -89.75) -> (36.8693, -103.75)
  arc A252 (30.3693, -89.25) -> (29.8693, -89.75) centre (30.3693, -89.75) ccw
  arc A253 (36.8693, -89.75) -> (36.3693, -89.25) centre (36.3693, -89.75) ccw
  arc A254 (29.8693, -103.75) -> (30.3693, -104.25) centre (30.3693, -103.75) ccw
  arc A255 (36.3693, -104.25) -> (36.8693, -103.75) centre (36.3693, -103.75) ccw
  line L260 (45.8875, -88.25) -> (58.8875, -88.25)
  line L261 (45.8875, -102.25) -> (58.8875, -102.25)
  line L262 (45.3875, -88.75) -> (45.3875, -101.75)
  line L263 (59.3875, -88.75) -> (59.3875, -101.75)
  arc A256 (45.8875, -88.25) -> (45.3875, -88.75) centre (45.8875, -88.75) ccw
  arc A257 (59.3875, -88.75) -> (58.8875, -88.25) centre (58.8875, -88.75) ccw
  arc A258 (45.3875, -101.75) -> (45.8875, -102.25) centre (45.8875, -101.75) ccw
  arc A259 (58.8875, -102.25) -> (59.3875, -101.75) centre (58.8875, -101.75) ccw
  line L264 (64.9375, -88.25) -> (77.9375, -88.25)
  line L265 (64.9375, -102.25) -> (77.9375, -102.25)
  line L266 (64.4375, -88.75) -> (64.4375, -101.75)
  line L267 (78.4375, -88.75) -> (78.4375, -101.75)
  arc A260 (64.9375, -88.25) -> (64.4375, -88.75) centre (64.9375, -88.75) ccw
  arc A261 (78.4375, -88.75) -> (77.9375, -88.25) centre (77.9375, -88.75) ccw
  arc A262 (64.4375, -101.75) -> (64.9375, -102.25) centre (64.9375, -101.75) ccw
  arc A263 (77.9375, -102.25) -> (78.4375, -101.75) centre (77.9375, -101.75) ccw
  line L268 (83.9875, -88.25) -> (96.9875, -88.25)
  line L269 (83.9875, -102.25) -> (96.9875, -102.25)
  line L270 (83.4875, -88.75) -> (83.4875, -101.75)
  line L271 (97.4875, -88.75) -> (97.4875, -101.75)
  arc A264 (83.9875, -88.25) -> (83.4875, -88.75) centre (83.9875, -88.75) ccw
  arc A265 (97.4875, -88.75) -> (96.9875, -88.25) centre (96.9875, -88.75) ccw
  arc A266 (83.4875, -101.75) -> (83.9875, -102.25) centre (83.9875, -101.75) ccw
  arc A267 (96.9875, -102.25) -> (97.4875, -101.75) centre (96.9875, -101.75) ccw
  line L272 (103.0375, -88.25) -> (116.0375, -88.25)
  line L273 (103.0375, -102.25) -> (116.0375, -102.25)
  line L274 (102.5375, -88.75) -> (102.5375, -101.75)
  line L275 (116.5375, -88.75) -> (116.5375, -101.75)
  arc A268 (103.0375, -88.25) -> (102.5375, -88.75) centre (103.0375, -88.75) ccw
  arc A269 (116.5375, -88.75) -> (116.0375, -88.25) centre (116.0375, -88.75) ccw
  arc A270 (102.5375, -101.75) -> (103.0375, -102.25) centre (103.0375, -101.75) ccw
  arc A271 (116.0375, -102.25) -> (116.5375, -101.75) centre (116.0375, -101.75) ccw
  line L276 (122.0875, -88.25) -> (135.0875, -88.25)
  line L277 (122.0875, -102.25) -> (135.0875, -102.25)
  line L278 (121.5875, -88.75) -> (121.5875, -101.75)
  line L279 (135.5875, -88.75) -> (135.5875, -101.75)
  arc A272 (122.0875, -88.25) -> (121.5875, -88.75) centre (122.0875, -88.75) ccw
  arc A273 (135.5875, -88.75) -> (135.0875, -88.25) centre (135.0875, -88.75) ccw
  arc A274 (121.5875, -101.75) -> (122.0875, -102.25) centre (122.0875, -101.75) ccw
  arc A275 (135.0875, -102.25) -> (135.5875, -101.75) centre (135.0875, -101.75) ccw
  line L280 (141.1375, -88.25) -> (154.1375, -88.25)
  line L281 (141.1375, -102.25) -> (154.1375, -102.25)
  line L282 (140.6375, -88.75) -> (140.6375, -101.75)
  line L283 (154.6375, -88.75) -> (154.6375, -101.75)
  arc A276 (141.1375, -88.25) -> (140.6375, -88.75) centre (141.1375, -88.75) ccw
  arc A277 (154.6375, -88.75) -> (154.1375, -88.25) centre (154.1375, -88.75) ccw
  arc A278 (140.6375, -101.75) -> (141.1375, -102.25) centre (141.1375, -101.75) ccw
  arc A279 (154.1375, -102.25) -> (154.6375, -101.75) centre (154.1375, -101.75) ccw
  line L284 (160.1875, -88.25) -> (173.1875, -88.25)
  line L285 (160.1875, -102.25) -> (173.1875, -102.25)
  line L286 (159.6875, -88.75) -> (159.6875, -101.75)
  line L287 (173.6875, -88.75) -> (173.6875, -101.75)
  arc A280 (160.1875, -88.25) -> (159.6875, -88.75) centre (160.1875, -88.75) ccw
  arc A281 (173.6875, -88.75) -> (173.1875, -88.25) centre (173.1875, -88.75) ccw
  arc A282 (159.6875, -101.75) -> (160.1875, -102.25) centre (160.1875, -101.75) ccw
  arc A283 (173.1875, -102.25) -> (173.6875, -101.75) centre (173.1875, -101.75) ccw
  line L288 (179.2375, -88.25) -> (192.2375, -88.25)
  line L289 (179.2375, -102.25) -> (192.2375, -102.25)
  line L290 (178.7375, -88.75) -> (178.7375, -101.75)
  line L291 (192.7375, -88.75) -> (192.7375, -101.75)
  arc A284 (179.2375, -88.25) -> (178.7375, -88.75) centre (179.2375, -88.75) ccw
  arc A285 (192.7375, -88.75) -> (192.2375, -88.25) centre (192.2375, -88.75) ccw
  arc A286 (178.7375, -101.75) -> (179.2375, -102.25) centre (179.2375, -101.75) ccw
  arc A287 (192.2375, -102.25) -> (192.7375, -101.75) centre (192.2375, -101.75) ccw
  line L292 (198.2875, -88.25) -> (211.2875, -88.25)
  line L293 (198.2875, -102.25) -> (211.2875, -102.25)
  line L294 (197.7875, -88.75) -> (197.7875, -101.75)
  line L295 (211.7875, -88.75) -> (211.7875, -101.75)
  arc A288 (198.2875, -88.25) -> (197.7875, -88.75) centre (198.2875, -88.75) ccw
  arc A289 (211.7875, -88.75) -> (211.2875, -88.25) centre (211.2875, -88.75) ccw
  arc A290 (197.7875, -101.75) -> (198.2875, -102.25) centre (198.2875, -101.75) ccw
  arc A291 (211.2875, -102.25) -> (211.7875, -101.75) centre (211.2875, -101.75) ccw
  line L296 (217.3375, -88.25) -> (230.3375, -88.25)
  line L297 (217.3375, -102.25) -> (230.3375, -102.25)
  line L298 (216.8375, -88.75) -> (216.8375, -101.75)
  line L299 (230.8375, -88.75) -> (230.8375, -101.75)
  arc A292 (217.3375, -88.25) -> (216.8375, -88.75) centre (217.3375, -88.75) ccw
  arc A293 (230.8375, -88.75) -> (230.3375, -88.25) centre (230.3375, -88.75) ccw
  arc A294 (216.8375, -101.75) -> (217.3375, -102.25) centre (217.3375, -101.75) ccw
  arc A295 (230.3375, -102.25) -> (230.8375, -101.75) centre (230.3375, -101.75) ccw
  line L300 (243.5313, -88.25) -> (256.5313, -88.25)
  line L301 (243.5313, -102.25) -> (256.5313, -102.25)
  line L302 (243.0312, -88.75) -> (243.0312, -101.75)
  line L303 (257.0312, -88.75) -> (257.0312, -101.75)
  arc A296 (243.5313, -88.25) -> (243.0313, -88.75) centre (243.5313, -88.75) ccw
  arc A297 (257.0312, -88.75) -> (256.5312, -88.25) centre (256.5312, -88.75) ccw
  arc A298 (243.0313, -101.75) -> (243.5313, -102.25) centre (243.5313, -101.75) ccw
  arc A299 (256.5312, -102.25) -> (257.0312, -101.75) centre (256.5312, -101.75) ccw
  line L304 (270.9156, -88.25) -> (283.9156, -88.25)
  line L305 (270.9156, -102.25) -> (283.9156, -102.25)
  line L306 (270.4156, -88.75) -> (270.4156, -101.75)
  line L307 (284.4156, -88.75) -> (284.4156, -101.75)
  arc A300 (270.9156, -88.25) -> (270.4156, -88.75) centre (270.9156, -88.75) ccw
  arc A301 (284.4156, -88.75) -> (283.9156, -88.25) centre (283.9156, -88.75) ccw
  arc A302 (270.4156, -101.75) -> (270.9156, -102.25) centre (270.9156, -101.75) ccw
  arc A303 (283.9156, -102.25) -> (284.4156, -101.75) centre (283.9156, -101.75) ccw
  line L308 (291.1562, -88.25) -> (304.1562, -88.25)
  line L309 (291.1562, -102.25) -> (304.1562, -102.25)
  line L310 (290.6562, -88.75) -> (290.6562, -101.75)
  line L311 (304.6562, -88.75) -> (304.6562, -101.75)
  arc A304 (291.1562, -88.25) -> (290.6562, -88.75) centre (291.1562, -88.75) ccw
  arc A305 (304.6562, -88.75) -> (304.1562, -88.25) centre (304.1562, -88.75) ccw
  arc A306 (290.6562, -101.75) -> (291.1562, -102.25) centre (291.1562, -101.75) ccw
  arc A307 (304.1562, -102.25) -> (304.6562, -101.75) centre (304.1562, -101.75) ccw
  line L312 (5.4062, -107.3) -> (18.4063, -107.3)
  line L313 (5.4062, -121.3) -> (18.4063, -121.3)
  line L314 (4.9062, -107.8) -> (4.9062, -120.8)
  line L315 (18.9062, -107.8) -> (18.9062, -120.8)
  arc A308 (5.4062, -107.3) -> (4.9062, -107.8) centre (5.4062, -107.8) ccw
  arc A309 (18.9062, -107.8) -> (18.4062, -107.3) centre (18.4062, -107.8) ccw
  arc A310 (4.9062, -120.8) -> (5.4062, -121.3) centre (5.4062, -120.8) ccw
  arc A311 (18.4062, -121.3) -> (18.9063, -120.8) centre (18.4062, -120.8) ccw
  line L316 (29.2188, -107.3) -> (42.2188, -107.3)
  line L317 (29.2188, -121.3) -> (42.2188, -121.3)
  line L318 (28.7188, -107.8) -> (28.7188, -120.8)
  line L319 (42.7188, -107.8) -> (42.7188, -120.8)
  arc A312 (29.2188, -107.3) -> (28.7187, -107.8) centre (29.2188, -107.8) ccw
  arc A313 (42.7188, -107.8) -> (42.2188, -107.3) centre (42.2188, -107.8) ccw
  arc A314 (28.7188, -120.8) -> (29.2188, -121.3) centre (29.2188, -120.8) ccw
  arc A315 (42.2188, -121.3) -> (42.7188, -120.8) centre (42.2188, -120.8) ccw
  line L320 (53.0313, -107.3) -> (66.0312, -107.3)
  line L321 (53.0313, -121.3) -> (66.0312, -121.3)
  line L322 (52.5313, -107.8) -> (52.5313, -120.8)
  line L323 (66.5312, -107.8) -> (66.5312, -120.8)
  arc A316 (53.0313, -107.3) -> (52.5312, -107.8) centre (53.0313, -107.8) ccw
  arc A317 (66.5312, -107.8) -> (66.0312, -107.3) centre (66.0312, -107.8) ccw
  arc A318 (52.5313, -120.8) -> (53.0313, -121.3) centre (53.0313, -120.8) ccw
  arc A319 (66.0312, -121.3) -> (66.5312, -120.8) centre (66.0312, -120.8) ccw
  line L324 (124.4688, -107.3) -> (137.4688, -107.3)
  line L325 (124.4688, -121.3) -> (137.4688, -121.3)
  line L326 (123.9688, -107.8) -> (123.9688, -120.8)
  line L327 (137.9688, -107.8) -> (137.9688, -120.8)
  arc A320 (124.4688, -107.3) -> (123.9688, -107.8) centre (124.4688, -107.8) ccw
  arc A321 (137.9688, -107.8) -> (137.4688, -107.3) centre (137.4688, -107.8) ccw
  arc A322 (123.9688, -120.8) -> (124.4688, -121.3) centre (124.4688, -120.8) ccw
  arc A323 (137.4688, -121.3) -> (137.9688, -120.8) centre (137.4688, -120.8) ccw
  line L328 (77.9688, -108.3) -> (83.9688, -108.3)
  line L329 (77.9688, -123.3) -> (83.9688, -123.3)
  line L330 (77.4688, -108.8) -> (77.4688, -122.8)
  line L331 (84.4688, -108.8) -> (84.4688, -122.8)
  arc A324 (77.9688, -108.3) -> (77.4688, -108.8) centre (77.9688, -108.8) ccw
  arc A325 (84.4688, -108.8) -> (83.9688, -108.3) centre (83.9688, -108.8) ccw
  arc A326 (77.4688, -122.8) -> (77.9688, -123.3) centre (77.9688, -122.8) ccw
  arc A327 (83.9688, -123.3) -> (84.4687, -122.8) centre (83.9688, -122.8) ccw
  line L332 (177.9688, -108.3) -> (183.9688, -108.3)
  line L333 (177.9688, -123.3) -> (183.9688, -123.3)
  line L334 (177.4688, -108.8) -> (177.4688, -122.8)
  line L335 (184.4688, -108.8) -> (184.4688, -122.8)
  arc A328 (177.9688, -108.3) -> (177.4688, -108.8) centre (177.9688, -108.8) ccw
  arc A329 (184.4688, -108.8) -> (183.9688, -108.3) centre (183.9688, -108.8) ccw
  arc A330 (177.4688, -122.8) -> (177.9688, -123.3) centre (177.9688, -122.8) ccw
  arc A331 (183.9688, -123.3) -> (184.4688, -122.8) centre (183.9688, -122.8) ccw
  line L336 (193.525, -107.3) -> (206.525, -107.3)
  line L337 (193.525, -121.3) -> (206.525, -121.3)
  line L338 (193.025, -107.8) -> (193.025, -120.8)
  line L339 (207.025, -107.8) -> (207.025, -120.8)
  arc A332 (193.525, -107.3) -> (193.025, -107.8) centre (193.525, -107.8) ccw
  arc A333 (207.025, -107.8) -> (206.525, -107.3) centre (206.525, -107.8) ccw
  arc A334 (193.025, -120.8) -> (193.525, -121.3) centre (193.525, -120.8) ccw
  arc A335 (206.525, -121.3) -> (207.025, -120.8) centre (206.525, -120.8) ccw
  line L340 (212.575, -107.3) -> (225.575, -107.3)
  line L341 (212.575, -121.3) -> (225.575, -121.3)
  line L342 (212.075, -107.8) -> (212.075, -120.8)
  line L343 (226.075, -107.8) -> (226.075, -120.8)
  arc A336 (212.575, -107.3) -> (212.075, -107.8) centre (212.575, -107.8) ccw
  arc A337 (226.075, -107.8) -> (225.575, -107.3) centre (225.575, -107.8) ccw
  arc A338 (212.075, -120.8) -> (212.575, -121.3) centre (212.575, -120.8) ccw
  arc A339 (225.575, -121.3) -> (226.075, -120.8) centre (225.575, -120.8) ccw
  line L344 (231.625, -107.3) -> (244.625, -107.3)
  line L345 (231.625, -121.3) -> (244.625, -121.3)
  line L346 (231.125, -107.8) -> (231.125, -120.8)
  line L347 (245.125, -107.8) -> (245.125, -120.8)
  arc A340 (231.625, -107.3) -> (231.125, -107.8) centre (231.625, -107.8) ccw
  arc A341 (245.125, -107.8) -> (244.625, -107.3) centre (244.625, -107.8) ccw
  arc A342 (231.125, -120.8) -> (231.625, -121.3) centre (231.625, -120.8) ccw
  arc A343 (244.625, -121.3) -> (245.125, -120.8) centre (244.625, -120.8) ccw
  line L348 (250.675, -107.3) -> (263.675, -107.3)
  line L349 (250.675, -121.3) -> (263.675, -121.3)
  line L350 (250.175, -107.8) -> (250.175, -120.8)
  line L351 (264.175, -107.8) -> (264.175, -120.8)
  arc A344 (250.675, -107.3) -> (250.175, -107.8) centre (250.675, -107.8) ccw
  arc A345 (264.175, -107.8) -> (263.675, -107.3) centre (263.675, -107.8) ccw
  arc A346 (250.175, -120.8) -> (250.675, -121.3) centre (250.675, -120.8) ccw
  arc A347 (263.675, -121.3) -> (264.175, -120.8) centre (263.675, -120.8) ccw
  line L352 (270.9156, -107.3) -> (283.9156, -107.3)
  line L353 (270.9156, -121.3) -> (283.9156, -121.3)
  line L354 (270.4156, -107.8) -> (270.4156, -120.8)
  line L355 (284.4156, -107.8) -> (284.4156, -120.8)
  arc A348 (270.9156, -107.3) -> (270.4156, -107.8) centre (270.9156, -107.8) ccw
  arc A349 (284.4156, -107.8) -> (283.9156, -107.3) centre (283.9156, -107.8) ccw
  arc A350 (270.4156, -120.8) -> (270.9156, -121.3) centre (270.9156, -120.8) ccw
  arc A351 (283.9156, -121.3) -> (284.4156, -120.8) centre (283.9156, -120.8) ccw
  line L356 (291.1562, -107.3) -> (304.1562, -107.3)
  line L357 (291.1562, -121.3) -> (304.1562, -121.3)
  line L358 (290.6562, -107.8) -> (290.6562, -120.8)
  line L359 (304.6562, -107.8) -> (304.6562, -120.8)
  arc A352 (291.1562, -107.3) -> (290.6562, -107.8) centre (291.1562, -107.8) ccw
  arc A353 (304.6562, -107.8) -> (304.1562, -107.3) centre (304.1562, -107.8) ccw
  arc A354 (290.6562, -120.8) -> (291.1562, -121.3) centre (291.1562, -120.8) ccw
  arc A355 (304.1562, -121.3) -> (304.6562, -120.8) centre (304.1562, -120.8) ccw
  line L360 (304.6562, -38.1) -> (318.4436, -38.1) construction
  line L361 (2.525, -14.287) -> (-11.2624, -14.287) construction
  line L362 (9.525, -7.287) -> (9.525, 12.475) construction
  circle A356 centre (-7.7624, 8.975) radius 1.7
  line L363 (-7.7624, 8.975) -> (-7.7624, 12.475) construction
  line L364 (-7.7624, 8.975) -> (-11.2624, 8.975) construction
  line L365 (153.5906, 12.475) -> (153.5906, 3.2274) construction
  line L366 (-11.2624, -61.269) -> (-2.7536, -61.269) construction
  circle A357 centre (314.9436, 8.975) radius 1.7
  circle A358 centre (-7.7624, -131.513) radius 1.7
  circle A359 centre (314.9436, -131.513) radius 1.7
  line L367 (54.625, -14.287) -> (59.675, -14.287) construction
  line L368 (73.675, -14.287) -> (78.725, -14.287) construction
  line L369 (92.725, -14.287) -> (97.775, -14.287) construction
  line L370 (140.3501, -14.287) -> (145.4001, -14.287) construction
  line L371 (159.4001, -14.287) -> (164.4501, -14.287) construction
  line L372 (178.4501, -14.287) -> (183.5001, -14.287) construction
  line L373 (226.0752, -14.287) -> (231.1252, -14.287) construction
  line L374 (245.1252, -14.287) -> (250.1752, -14.287) construction
  line L375 (264.1753, -14.287) -> (269.2253, -14.287) construction
  line L376 (16.525, -38.1) -> (21.575, -38.1) construction
  line L377 (197.5001, -14.287) -> (212.0752, -14.287) construction
  line L378 (111.775, -14.287) -> (126.3501, -14.287) construction
  line L379 (285.7503, -4.762) -> (266.7003, -4.762) construction
  line L380 (266.7003, -4.762) -> (266.7003, -23.812) construction
  line L381 (266.7003, -23.812) -> (285.7503, -23.812) construction
  line L382 (285.7503, -23.812) -> (285.7503, -4.762) construction
  line L383 (285.7503, -4.762) -> (266.7003, -23.812) construction
  line L384 (266.7003, -4.762) -> (285.7503, -23.812) construction
  line L385 (307.1812, -28.575) -> (288.1312, -28.575) construction
  line L386 (288.1313, -28.575) -> (288.1313, -47.625) construction
  line L387 (288.1313, -47.625) -> (307.1813, -47.625) construction
  line L388 (307.1812, -47.625) -> (307.1812, -28.575) construction
  line L389 (307.1812, -28.575) -> (288.1312, -47.625) construction
  line L390 (288.1313, -28.575) -> (307.1813, -47.625) construction
  line L391 (19.05, -4.762) -> (0, -4.762) construction
  line L392 (0, -4.762) -> (0, -23.812) construction
  line L393 (0, -23.812) -> (19.05, -23.812) construction
  line L394 (19.05, -23.812) -> (19.05, -4.762) construction
  line L395 (19.05, -4.762) -> (0, -23.812) construction
  line L396 (0, -4.762) -> (19.05, -23.812) construction
  line L397 (0, -28.575) -> (19.05, -28.575) construction
  line L398 (19.05, -28.575) -> (19.05, -47.625) construction
  line L399 (19.05, -47.625) -> (0, -47.625) construction
  line L400 (0, -47.625) -> (0, -28.575) construction
  line L401 (0, -28.575) -> (19.05, -47.625) construction
  line L402 (19.05, -28.575) -> (0, -47.625) construction
  circle A360 centre (297.6562, -14.287) radius 9.2
  point P0 (276.2253, -14.287)
  point P1 (276.2253, -14.287)
  point P2 (283.2253, -14.287)
  point P3 (297.6562, -38.1)
  point P4 (297.6562, -31.1)
  point P5 (297.6562, -38.1)
  point P6 (276.2253, -7.287)
  point P7 (9.525, -14.287)
  point P8 (9.525, -31.1)
  point P9 (2.525, -38.1)
  point P10 (9.525, -38.1)
  dimension "d28" = 147.488
  dimension "d29" = 329.706
  dimension "d32" = 3.4
  dimension "d33" = 3.5
  dimension "d35" = 13.713
  dimension "d39" = 19.05
  dimension "d40" = 19.05
  dimension "d41" = 2.381
  dimension "d42" = 4.763
  dimension "d43" = 18.4
  constraint horizontal L0
  constraint vertical L1
  constraint horizontal L2
  constraint vertical L3
  constraint midpoint L123 L360.start